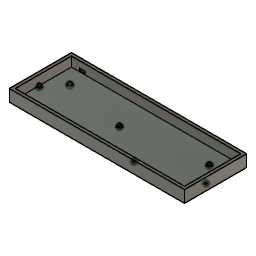
Case (Autodesk Fusion 360 design; units mm, degrees)
Autodesk Fusion 360 part; units mm, degrees
sketch "Body" plane through (0, 0, 0) normal (0, 0, 1) x (1, 0, 0)
  line L0 (147.5, -52.3) -> (-147.5, -52.3)
  line L1 (-147.5, -52.3) -> (-147.5, 52.3)
  line L2 (-147.5, 52.3) -> (147.5, 52.3)
  line L3 (147.5, 52.3) -> (147.5, -52.3)
  line L4 (147.5, -52.3) -> (-147.5, 52.3) construction
  line L5 (-147.5, -52.3) -> (147.5, 52.3) construction
  dimension "d15" = 295
  dimension "d16" = 104.6
  constraint horizontal L0
  constraint perpendicular L0 L1
  constraint parallel L0 L2
  constraint parallel L1 L3
  constraint coincident L4 origin
  constraint coincident L5 origin
  measures "d15" distance of L1.end L2.end
  measures "d16" distance of L0.end L1.end
extrude "Extrude3" add sketch "Body" along normal blind 20
sketch "Walls" plane through (0, 0, 20) normal (0, 0, 1) x (-1, 0, 0)
  line L0 (-147.5, -52.3) -> (147.5, -52.3)
  line L1 (147.5, -52.3) -> (147.5, 52.3)
  line L2 (147.5, 52.3) -> (-147.5, 52.3)
  line L3 (-147.5, 52.3) -> (-147.5, -52.3)
  line L4 (142.5, 47.3) -> (-142.5, 47.3)
  line L5 (-142.5, 47.3) -> (-142.5, -47.3)
  line L6 (-142.5, -47.3) -> (142.5, -47.3)
  line L7 (142.5, -47.3) -> (142.5, 47.3)
  dimension "d19" = -5
extrude "Extrude4" cut sketch "Walls" against normal up to surface (16 mm away) contours L4 L5 L6 L7
sketch "Screws" plane through (0, 0, 4) normal (0, 0, 1) x (-1, 0, 0)
  line L0 (142.5, 47.3) -> (-142.5, 47.3)
  line L1 (-142.5, 47.3) -> (-142.5, -47.3)
  line L2 (-142.5, -47.3) -> (142.5, -47.3)
  line L3 (142.5, -47.3) -> (142.5, 47.3)
  circle A0 centre (117.3, -19.4) radius 1.625
  circle A1 centre (140.5, 9.2) radius 1.625
  circle A2 centre (14.5, -0.3) radius 1.625
  circle A3 centre (-48, 37.9) radius 1.625
  circle A4 centre (-117.55, -19.4) radius 1.625
  circle A5 centre (-140.5, 9.2) radius 1.625
  circle A6 centre (140.5, 9.2) radius 0.625
  circle A7 centre (117.3, -19.4) radius 0.625
  circle A8 centre (14.5, -0.3) radius 0.625
  circle A9 centre (-48, 37.9) radius 0.625
  circle A10 centre (-117.55, -19.4) radius 0.625
  circle A11 centre (-140.5, 9.2) radius 0.625
  point P0 (117.3, -19.4)
  dimension "d32" = 3.25
  dimension "d33" = 27.9
  dimension "d34" = 25.2
  dimension "d35" = 3.25
  dimension "d36" = 2
  dimension "d37" = 56.5
  dimension "d38" = 3.25
  dimension "d39" = 128
  dimension "d40" = 47
  dimension "d41" = 3.25
  dimension "d42" = 85.2
  dimension "d43" = 190.5
  dimension "d44" = 3.25
  dimension "d45" = 27.9
  dimension "d46" = 24.95
  dimension "d47" = 3.25
  dimension "d48" = 56.5
  dimension "d49" = 2
  dimension "d57" = -1
  dimension "d58" = -1
  dimension "d59" = -1
  dimension "d60" = -1
  dimension "d61" = -1
  dimension "d62" = -1
  measures "d32" diameter of A0
  measures "d33" distance of L2 P0
  measures "d34" distance of L3 P0
  measures "d35" diameter of A1
  measures "d36" distance of L3 A1.centre
  measures "d37" distance of L2 A1.centre
  measures "d38" diameter of A2
  measures "d39" distance of L3 A2.centre
  measures "d40" distance of L2 A2.centre
  measures "d41" diameter of A3
  measures "d42" distance of L2 A3.centre
  measures "d43" distance of L3 A3.centre
  measures "d44" diameter of A4
  measures "d45" distance of L2 A4.centre
  measures "d46" distance of L1 A4.centre
  measures "d47" diameter of A5
  measures "d48" distance of L2 A5.centre
  measures "d49" distance of L1 A5.centre
extrude "Extrude9" add sketch "Screws" along normal blind 5 contours A0 | A1 | A2 | A3 | A4 | A5
fillet "Fillet1" [suppressed]
thread "Thread2" [suppressed]
sketch "Sketch13" plane through (0, 47.3, 0) normal (0, -1, 0) x (1, 0, 0)
  line L0 (-142.5, 4) -> (142.5, 4)
  line L1 (142.5, 4) -> (142.5, 20)
  line L2 (142.5, 20) -> (-142.5, 20)
  line L3 (-142.5, 20) -> (-142.5, 4)
  line L4 (-119.83, 9) -> (-128.77, 9)
  line L5 (-128.77, 9) -> (-128.77, 5.69)
  line L6 (-128.77, 5.69) -> (-119.83, 5.69)
  line L7 (-119.83, 5.69) -> (-119.83, 9)
  line L8 (-119.83, 9) -> (-128.77, 5.69) construction
  line L9 (-128.77, 9) -> (-119.83, 5.69) construction
  line L10 (142.5, 4) -> (-142.5, 4)
  point P0 (-124.3, 7.345)
  dimension "d65" = 8.94
  dimension "d66" = 3.31
  dimension "d67" = 18.2
  dimension "d71" = 5
  constraint horizontal L4
  constraint perpendicular L4 L5
  constraint parallel L4 L6
  constraint parallel L5 L7
  constraint coincident L8 P0
  constraint coincident L9 P0
  measures "d65" distance of L5.end L6.end
  measures "d66" distance of L4.end L5.end
  measures "d67" distance of L3 P0
  measures "d71" distance of L0 L4
extrude "Extrude10" cut sketch "Sketch13" against normal up to surface (5 mm away) contours L4 L5 L6 L7
fillet "Fillet3" [suppressed]
equation "d15 = 285 mm + 10 mm"
equation "d16 = 94.6 mm + 10 mm"
equation "d32 = 2 mm + 1.25 mm"
equation "d67 = 25.2 mm - 7 mm"
equation "d73 = ( 3.31 / 2 ) * 1 mm"
